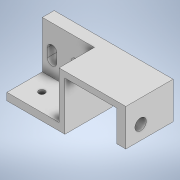
# Autodesk Inventor part: Compliant_plate
Saved by Autodesk Inventor 2022 (Build 260153000, 153)
## iProperties
Created: 2021-07-31
Part Number: Compliant_plate
Material: Generic
Document SubType Name: Modeling
Designer: exllu
Density: 1 g/cm^3
Appearance: Default
Mass: 4.01224 g
Surface Area: 39.1309 cm^2
Volume: 4.01224 cm^3
Author: exllu
Autodesk Inventor part; units mm, degrees
ref_plane "YZ Plane" through (0, 0, 0) normal (1, 0, 0) x (0, 1, 0)
ref_plane "XZ Plane" through (0, 0, 0) normal (0, 1, 0) x (-1, 0, 0)
ref_plane "XY Plane" through (0, 0, 0) normal (0, 0, 1) x (1, 0, 0)
sketch "Sketch1" plane through (0, 0, 0) normal (0, 0, 1) x (1, 0, 0)
  line L0 (0, 0) -> (49.1, 0)
  line L1 (49.1, 0) -> (49.1, 12.5)
  line L2 (49.1, 12.5) -> (0, 12.5)
  line L3 (0, 12.5) -> (0, 0)
  line L4 (0, 0) -> (49.1, 0)
  line L5 (49.1, 0) -> (49.1, 12.5)
  dimension "d0" = 49.1
  dimension "d1" = 12.5
  constraints: 12 end point, 2 horizontal, 2 parallel, 1 perpendicular, 1 vertical
  measures "d0" distance of L0.start L0.end
  measures "d1" distance of L0.end L1.end
extrude "Extrusion1" add sketch "Sketch1" along normal blind 14
sketch "Sketch2" plane through (0, 0, 0) normal (-1, 0, 0) x (0, 0, 1)
  line L0 (0, 0) -> (2, 0)
  line L1 (2, 0) -> (2, 5)
  line L2 (2, 5) -> (0, 5)
  line L3 (0, 5) -> (0, 0)
  dimension "d4" = 2
  dimension "d5" = 5
  constraints: 8 end point, 2 parallel, 1 horizontal, 1 perpendicular
  measures "d4" distance of L2.end L1.end
  measures "d5" distance of L1.end L0.end
sketch "Sketch3" plane through (0, 0, 14) normal (0, 0, 1) x (1, 0, 0)
  line L0 (0, 12.5) -> (0, 0) projected
  line L1 (49.1, 0) -> (49.1, 12.5) projected
  line L2 (0, 0) -> (49.1, 0)
  line L3 (49.1, 0) -> (47.6, 0)
  line L4 (0, 0) -> (49.1, 0) projected
  line L5 (47.6, 0) -> (47.6, 11.5)
  line L6 (49.1, 12.5) -> (0, 12.5) projected
  line L7 (47.6, 11.5) -> (19.65, 11.5)
  line L8 (19.65, 11.5) -> (19.65, 0)
  dimension "d8" = 1.5
  dimension "d9" = 11.5
  dimension "d10" = 27.95
  constraints: 10 end point, 3 perpendicular, 2 point on line, 1 horizontal
  measures "d8" distance of L1.start L3.end
  measures "d9" distance of L3.end L5.end
  measures "d10" distance of L5.end L7.end
extrude "Extrusion3" cut sketch "Sketch3" against normal blind 13 contours L8 L7 L5 L2
sketch "Sketch4" plane through (0, 0, 14) normal (-1, 0, 0) x (0, 0, 1)
  line L0 (0, 12.5) -> (0, 0) projected
  line L1 (0, 0) -> (0, 2)
  line L2 (0, 2) -> (0, 12.5)
  line L3 (0, 2) -> (-10, 2)
  line L4 (-12, 5) -> (-12, 0) projected
  line L5 (-10, 2) -> (-10, 12.5)
  line L6 (-14, 12.5) -> (0, 12.5) projected
  line L7 (-10, 12.5) -> (0, 12.5)
  point P0 (-14, 0)
  dimension "d13" = 2
  dimension "d14" = 10
  constraints: 10 end point, 2 collinear, 1 parallel, 1 perpendicular, 1 point on line
  measures "d13" distance of L0.end L1.end
  measures "d14" distance of L1.end L3.end
extrude "Extrusion4" cut sketch "Sketch4" against normal blind 17.65
sketch "Sketch5" plane through (0, 2, 14) normal (0, 1, 0) x (1, 0, 0)
  line L0 (17.65, 0) -> (0, 0) projected
  line L1 (0, 0) -> (5.825, 0)
  line L2 (5.825, 0) -> (5.825, 6)
  line L3 (5.825, 6) -> (13.825, 6)
  circle A0 centre (5.825, 6) radius 1.05
  circle A1 centre (13.825, 6) radius 1.05
  point P0 (0, 14)
  dimension "d18" = 5.825
  dimension "d19" = 6
  dimension "d20" = 8
  dimension "d21" = 2.1
  dimension "d22" = 2.1
  constraints: 6 end point, 4 coincident, 2 centre point, 1 horizontal, 1 perpendicular, 1 point on line
  measures "d18" distance of L0.end L1.end
  measures "d19" distance of L1.end L2.end
  measures "d20" distance of L2.end L3.end
  measures "d21" diameter of A0
  measures "d22" diameter of A1
hole "Hole1" at (5.825, 2, 8) at (13.825, 2, 8) direction (0, -1, 0) diameter 2.1 depth 20 tip angle 118
sketch "Sketch6" plane through (0, 0, 0) normal (0, 0, -1) x (-1, 0, 0)
  line L0 (0, 12.5) -> (0, 8.5)
  line L1 (0, 8.5) -> (-3.3, 8.5)
  line L2 (-4.9, 8.5) -> (-11.3, 8.5)
  line L3 (-12.9, 8.5) -> (-28.3, 8.5)
  line L4 (-28.3, 9.8) -> (-28.3, 10.5)
  line L5 (-28.3, 9.2) -> (-28.3, 7.5)
  line L6 (-11.3, 8.5) -> (-11.3, 10.5)
  line L7 (-11.3, 10.5) -> (-11.3, 7.5)
  line L8 (-3.3, 8.5) -> (-3.3, 9.1)
  line L9 (-3.3, 10.5) -> (-3.3, 7.5)
  arc A0 (-29.9, 7.5) -> (-26.7, 7.5) centre (-28.3, 7.5) ccw
  arc A1 (-4.9, 7.5) -> (-1.7, 7.5) centre (-3.3, 7.5) ccw
  arc A2 (-1.7, 10.5) -> (-4.9, 10.5) centre (-3.3, 10.5) ccw
  line L10 (-26.7, 10.5) -> (-26.7, 7.5)
  line L11 (-29.9, 7.5) -> (-29.9, 10.5)
  line L12 (-12.9, 10.5) -> (-12.9, 7.5)
  line L13 (-9.7, 7.5) -> (-9.7, 10.5)
  line L14 (-4.9, 10.5) -> (-4.9, 7.5)
  line L15 (-1.7, 7.5) -> (-1.7, 10.5)
  arc A3 (-12.9, 7.5) -> (-9.7, 7.5) centre (-11.3, 7.5) ccw
  arc A4 (-9.7, 10.5) -> (-12.9, 10.5) centre (-11.3, 10.5) ccw
  arc A5 (-26.7, 10.5) -> (-29.9, 10.5) centre (-28.3, 10.5) ccw
  arc A6 (-29.1307, 9.5) -> (-28.3, 9.2) centre (-28.3, 10.5) ccw
  point P0 (0, 0)
  dimension "d30" = 4
  dimension "d31" = 3.3
  dimension "d32" = 8
  dimension "d33" = 17
  dimension "d47" = 2
  dimension "d48" = 1
  dimension "d49" = 2
  dimension "d50" = 3
  dimension "d51" = 2
  dimension "d52" = 3
  dimension "d53" = 3.2
  dimension "d55" = 3.2
  dimension "d56" = 3.2
  dimension "d134" = 1.6
  constraints: 32 end point, 15 point on circle, 9 coincident, 9 tangent, 7 centre point, 6 point on line, 4 vertical, 1 perpendicular
  measures "d30" distance of L0.start L0.end
  measures "d31" distance of L0.end L1.end
  measures "d32" distance of L1.end L2.end
  measures "d33" distance of L2.end L3.end
  measures "d47" distance of point (-28.3, 8.5) L4.end
  measures "d48" distance of point (-28.3, 8.5) L5.end
  measures "d49" distance of L6.start L6.end
  measures "d50" distance of L6.end L7.end
  measures "d51" distance of L8.start L9.start
  measures "d52" distance of L9.start L9.end
  measures "d53" diameter of A0
  measures "d55" diameter of A1
  measures "d56" diameter of A2
  measures "d134" radius of A4
sketch "Sketch7" plane through (0, 0, 14) normal (0, 0, 1) x (1, 0, 0)
  line L0 (0, 12.5) -> (0, 0) projected
  line L1 (19.65, 0) -> (19.65, 11.5) projected
  line L2 (0, 0) -> (19.65, 0)
  line L3 (19.65, 0) -> (19.65, 2)
  line L4 (19.65, 2) -> (0, 2)
  line L5 (0, 2) -> (0, 0)
  line L6 (17.65, 12.5) -> (15.65, 12.5) projected
  line L7 (19.65, 2) -> (17.65, 2)
  line L8 (17.65, 2) -> (17.65, 12.5)
  line L9 (17.65, 12.5) -> (19.65, 12.5)
  line L10 (19.65, 12.5) -> (19.65, 2)
  line L11 (49.1, 0) -> (49.1, 12.5) projected
  line L12 (17.65, 12.5) -> (49.1, 12.5)
  line L13 (49.1, 12.5) -> (49.1, 11.5)
  line L14 (47.6, 11.5) -> (19.65, 11.5)
  line L15 (17.65, 11.5) -> (17.65, 12.5)
  line L16 (47.6, 11.5) -> (47.6, 0) projected
  line L17 (47.6, 11.5) -> (47.6, 0)
  line L18 (47.6, 0) -> (49.1, 0)
  line L19 (49.1, 0) -> (49.1, 11.5)
  dimension "d41" = 2
  constraints: 30 end point, 7 parallel, 3 horizontal, 3 perpendicular, 3 point on line
  measures "d41" distance of L3.end L2.end
extrude "Extrusion5" add sketch "Sketch7" along normal blind 2
sketch "Sketch9" plane through (0, 0, 0) normal (-1, 0, 0) x (0, 0, 1)
  line L0 (0, 0) -> (16, 0) projected
  line L1 (1, 0) -> (1, 11.5) projected
  line L2 (0, 0) -> (1, 0)
  line L3 (1, 0) -> (1, 4)
  line L4 (1, 4) -> (0, 4)
  line L5 (0, 4) -> (0, 0)
  dimension "d44" = 4
  constraints: 8 end point, 2 parallel, 1 horizontal, 1 perpendicular, 1 point on line
  measures "d44" distance of L3.end L2.end
extrude "Extrusion6" cut sketch "Sketch9" against normal blind 100
sketch "Sketch11" plane through (0, 2, 4) normal (-1, 0, 0) x (0, 0, 1)
  line L0 (0, 0) -> (0, 10.5) projected
  line L1 (0, 0) -> (0, 2)
  line L2 (-4, 10.5) -> (-4, 2) projected
  line L3 (0, 2) -> (-4, 2)
  line L4 (-4, 2) -> (-6, 2)
  line L5 (-6, 2) -> (-6, 10.5)
  line L6 (-4, 10.5) -> (0, 10.5) projected
  line L7 (-6, 10.5) -> (-4, 10.5)
  line L8 (-4, 10.5) -> (-4, 2)
  point P0 (-4, -2)
  dimension "d61" = 2
  dimension "d62" = 4
  dimension "d63" = 2
  constraints: 12 end point, 2 perpendicular, 2 point on line
  measures "d61" distance of L0.start L1.end
  measures "d62" distance of L1.end L2.end
  measures "d63" distance of L2.end L4.end
extrude "Extrusion8" add sketch "Sketch11" against normal blind 49.1 contours L4 L5 L7 L2
extrude "Extrusion7" cut sketch "Sketch6" along normal blind 100 and the other way blind 50
sketch "Sketch12" plane through (0, 2, 4) normal (-1, 0, 0) x (0, 0, 1)
  line L0 (0, 0) -> (0, 10.5) projected
  line L1 (0, 0) -> (-3, 0)
  line L2 (-3, -2) -> (-3, 2) projected
  line L3 (-3, -2) -> (12, -2) projected
  line L4 (-3, -2) -> (-6, -2)
  line L5 (-3, 2) -> (-6, 2) projected
  line L6 (-6, -2) -> (-6, 2)
  line L7 (-6, 2) -> (-3, 2)
  line L8 (-3, 2) -> (-3, -2)
  point P0 (-4, -2)
  dimension "d68" = 3
  dimension "d69" = 4
  dimension "d70" = 90
  constraints: 10 end point, 1 horizontal, 1 midpoint, 1 perpendicular
  measures "d68" distance of L2.start L4.end
  measures "d69" distance of L4.end L5.end
  measures "d70" angle of L4 L6
extrude "Extrusion9" add sketch "Sketch12" against normal blind 49.1
sketch "Sketch13" plane through (47.6, 0, 1) normal (-1, 0, 0) x (0, 0, 1)
  line L0 (15, 0) -> (0, 0) projected
  line L1 (0, 11.5) -> (0, 0) projected
  line L2 (0, 0) -> (0, 11.5)
  line L3 (15, 11.5) -> (0, 11.5) projected
  line L4 (0, 11.5) -> (15, 11.5)
  line L5 (15, 11.5) -> (15, 0)
  line L6 (15, 0) -> (0, 0)
  point P0 (-1, 0)
  constraints: 8 end point, 2 collinear, 2 perpendicular
extrude "Extrusion10" add sketch "Sketch13" along normal blind 1
sketch "Sketch14" plane through (49.1, 0, 16) normal (1, 0, 0) x (0, 0, -1)
  line L0 (15, 0) -> (0, 0) projected
  line L1 (18, 12.5) -> (0, 12.5) projected
  line L2 (0, 0) -> (18, 0)
  line L3 (18, 0) -> (18, 12.5)
  line L4 (18, 12.5) -> (0, 12.5)
  line L5 (0, 12.5) -> (0, 0)
  point P0 (16, 0)
  constraints: 8 end point, 2 parallel, 1 horizontal, 1 perpendicular
extrude "Extrusion11" cut sketch "Sketch14" against normal blind 12.3
sketch "Sketch15" plane through (36.8, 0, 16) normal (1, 0, 0) x (0, 0, -1)
  line L0 (18, 12.5) -> (18, 0) projected
  line L1 (15, 0) -> (0, 0) projected
  line L2 (18, 12.5) -> (0, 12.5)
  line L3 (0, 12.5) -> (0, 0)
  line L4 (0, 0) -> (18, 0)
  line L5 (18, 0) -> (18, 12.5)
  point P0 (16, 0)
  point P1 (18, 0)
  constraints: 8 end point, 2 parallel, 1 horizontal, 1 perpendicular
extrude "Extrusion12" add sketch "Sketch15" along normal blind 2.5
sketch "Sketch17" plane through (0, 0, -2) normal (0, -1, 0) x (1, 0, 0)
  line L0 (39.3, 0) -> (39.3, 18) projected
  line L1 (39.3, 0) -> (39.3, 16)
  line L2 (39.3, 16) -> (36.8, 16)
  line L3 (36.8, 3) -> (36.8, 18) projected
  line L4 (36.8, 16) -> (36.8, 3)
  line L5 (19.65, 3) -> (36.8, 3) projected
  line L6 (36.8, 3) -> (19.65, 3)
  line L7 (19.65, 3) -> (19.65, 0)
  line L8 (0, 0) -> (39.3, 0) projected
  line L9 (19.65, 0) -> (39.3, 0)
  point P0 (0, 2)
  constraints: 12 end point, 3 collinear, 3 perpendicular
extrude "Extrusion14" cut sketch "Sketch17" against normal blind 5
sketch "Sketch18" plane through (36.8, 0, 16) normal (0, -1, 0) x (1, 0, 0)
  line L0 (2.5, 0) -> (-19.15, 0) projected
  line L1 (2.5, 0) -> (0, 0)
  line L2 (0, 0) -> (0, -2)
  line L3 (0, -2) -> (2.5, -2)
  line L4 (2.5, -2) -> (2.5, 0)
  point P0 (-36.8, -16)
  dimension "d84" = 2.5
  dimension "d85" = 2
  constraints: 8 end point, 2 parallel, 1 horizontal, 1 perpendicular
  measures "d84" distance of L3.end L2.end
  measures "d85" distance of L2.end L1.end
extrude "Extrusion15" cut sketch "Sketch18" against normal blind 5
sketch "Sketch19" plane through (19.65, 11.5, 1) normal (0, -1, 0) x (1, 0, 0)
  line L0 (0, 15) -> (0, 0) projected
  line L1 (0, 0) -> (0, 15)
  line L2 (0, 15) -> (17.15, 15)
  line L3 (19.65, 15) -> (-2, 15) projected
  line L4 (17.15, 15) -> (17.15, 0)
  line L5 (17.15, 0) -> (0, 0)
  point P0 (-19.65, -1)
  point P1 (0, 0)
  dimension "d88" = 17.15
  dimension "d89" = 15
  constraints: 8 end point, 2 perpendicular, 2 point on line, 1 collinear
  measures "d88" distance of L0.start L2.end
  measures "d89" distance of L2.end L4.end
extrude "Extrusion16" cut sketch "Sketch19" against normal blind 5
sketch "Sketch20" plane through (0, 12.5, 4) normal (0, 1, 0) x (1, 0, 0)
  line L0 (0, 6) -> (0, -12) projected
  line L1 (0, 6) -> (0, 0)
  line L2 (0, 6) -> (39.3, 6) projected
  line L3 (0, 6) -> (39.3, 6)
  line L4 (39.3, -12) -> (39.3, 6) projected
  line L5 (39.3, 6) -> (39.3, -12)
  line L6 (39.3, -12) -> (36.8, -12) projected
  line L7 (39.3, -12) -> (36.8, -12)
  line L8 (36.8, -12) -> (36.8, 3)
  line L9 (36.8, 3) -> (19.65, 3)
  line L10 (19.65, -12) -> (19.65, 3) projected
  line L11 (19.65, 3) -> (19.65, -12)
  line L12 (17.65, -12) -> (17.65, 0) projected
  line L13 (19.65, -12) -> (17.65, -12)
  line L14 (17.65, -12) -> (17.65, 0)
  line L15 (17.65, 0) -> (17.65, 6)
  point P0 (0, 4)
  dimension "d92" = 6
  constraints: 20 end point, 4 collinear, 3 perpendicular, 3 point on line, 1 horizontal
  measures "d92" distance of L0.start L1.end
extrude "Extrusion17" add sketch "Sketch20" along normal blind 4
sketch "Sketch21" plane through (0, 12.5, 4) normal (0, 1, 0) x (1, 0, 0)
  line L0 (0, -12) -> (0, 0) projected
  line L1 (0, 0) -> (17.65, 0)
  line L2 (17.65, 0) -> (17.65, 6)
  line L3 (17.65, 6) -> (0, 6)
  line L4 (0, 6) -> (0, 0)
  point P0 (0, 4)
  constraints: 8 end point, 2 parallel, 1 horizontal, 1 perpendicular
extrude "Extrusion18" add sketch "Sketch21" along normal blind 4
sketch "Sketch22" plane through (0, 16.5, 4) normal (0, 1, 0) x (1, 0, 0)
  line L0 (0, 6) -> (0, 0) projected
  line L1 (0, 0) -> (36.92, 0)
  line L2 (19.65, 3) -> (36.8, 3) projected
  line L3 (36.8, 3) -> (36.8, 0)
  line L4 (36.8, 3) -> (36.8, -12) projected
  line L5 (36.8, 0) -> (36.3, 0)
  line L6 (36.3, 0) -> (36.3, 3)
  point P0 (0, 4)
  dimension "d97" = 3
  dimension "d98" = 0.5
  constraints: 8 end point, 2 point on line, 1 horizontal, 1 perpendicular
  measures "d97" distance of L2.end L3.end
  measures "d98" distance of L3.end L5.end
extrude "Extrusion19" add sketch "Sketch22" against normal blind 11.5
sketch "Sketch23" plane through (36.8, 0, 16) normal (-1, 0, 0) x (0, 0, 1)
  line L0 (0, 0) -> (0, 5)
  line L1 (-12, 5) -> (0, 5) projected
  line L2 (0, 5) -> (-12, 5)
  line L3 (-12, 16.5) -> (-12, 5) projected
  line L4 (-12, 5) -> (-12, 16.5)
  line L5 (-12, 16.5) -> (0, 16.5)
  line L6 (0, 16.5) -> (0, 5)
  line L7 (0, 5) -> (0, 16.5) projected
  line L8 (0, 10.75) -> (-7, 10.75)
  circle A0 centre (-7, 10.75) radius 1.9304
  point P0 (-16, 0)
  dimension "d101" = 5
  dimension "d102" = 12
  dimension "d103" = 7
  dimension "d104" = 3.8608
  constraints: 12 end point, 3 perpendicular, 1 centre point, 1 coincident, 1 collinear, 1 horizontal, 1 midpoint, 1 vertical
  measures "d101" distance of L0.start L0.end
  measures "d102" distance of L0.end L1.start
  measures "d103" distance of L8.start L8.end
  measures "d104" diameter of A0
sketch "Sketch24" plane through (0, 16.5, 4) normal (0, 1, 0) x (1, 0, 0)
  line L0 (39.3, -12) -> (39.3, 6) projected
  line L1 (39.3, -12) -> (36.3, -12)
  line L2 (36.8, -12) -> (39.3, -12) projected
  line L3 (36.3, -12) -> (36.3, 0)
  line L4 (36.3, 0) -> (36.8, 0) projected
  line L5 (36.8, 0) -> (36.8, -12) projected
  line L6 (36.8, 0) -> (36.8, -12)
  point P0 (0, 4)
  dimension "d107" = 3
  constraints: 6 end point, 2 collinear, 1 perpendicular, 1 point on line
  measures "d107" distance of L0.start L1.end
extrude "Extrusion21" add sketch "Sketch24" against normal blind 11.5
extrude "Extrusion22" cut sketch "Sketch23" along normal mid plane 11.5 contours A0
sketch "Sketch25" plane through (0, 16.5, 4) normal (0, 1, 0) x (1, 0, 0)
  line L0 (17.65, -12) -> (0, -12) projected
  line L1 (39.3, 6) -> (0, 6) projected
  line L2 (0, -12) -> (39.3, -12)
  line L3 (39.3, -12) -> (39.3, 6)
  line L4 (39.3, 6) -> (0, 6)
  line L5 (0, 6) -> (0, -12)
  line L6 (0, 0) -> (17.65, 0) projected
  line L7 (17.65, 0) -> (0, 0)
  line L8 (0, 0) -> (0, -12)
  line L9 (0, -12) -> (17.65, -12)
  line L10 (17.65, -12) -> (17.65, 0)
  point P0 (0, 4)
  constraints: 16 end point, 4 parallel, 2 horizontal, 2 perpendicular
extrude "Extrusion23" add sketch "Sketch25" along normal blind 2 contours L10 L6 L5 L1 L3 L2
sketch "Sketch26" plane through (0, 0, 16) normal (0, 0, 1) x (1, 0, 0)
  line L0 (0, 18.5) -> (0, 0) projected
  line L1 (19.65, 0) -> (19.65, 16.5) projected
  line L2 (0, 0) -> (19.65, 0)
  line L3 (19.65, 5) -> (19.65, 16.5) projected
  line L4 (19.65, 0) -> (19.65, 16.5)
  line L5 (19.65, 16.5) -> (36.3, 16.5) projected
  line L6 (19.65, 16.5) -> (36.3, 16.5)
  line L7 (36.3, 16.5) -> (36.3, 5) projected
  line L8 (36.3, 16.5) -> (36.3, 5)
  line L9 (39.3, 5) -> (19.65, 5) projected
  line L10 (36.3, 5) -> (39.3, 5)
  line L11 (39.3, 18.5) -> (0, 18.5) projected
  line L12 (39.3, 5) -> (39.3, 18.5)
  line L13 (39.3, 18.5) -> (17.65, 18.5)
  line L14 (0, 2) -> (17.65, 2) projected
  line L15 (0, 0) -> (0, 2)
  line L16 (0, 2) -> (17.65, 2)
  line L17 (0, 2) -> (17.65, 2)
  line L18 (17.65, 2) -> (17.65, 18.5)
  line L19 (17.65, 18.5) -> (0, 18.5)
  line L20 (0, 18.5) -> (0, 2)
  dimension "d114" = 3
  dimension "d115" = 21.65
  constraints: 26 end point, 4 perpendicular, 3 collinear, 2 horizontal, 2 parallel, 1 point on line, 1 vertical
  measures "d114" distance of L7.end L9.start
  measures "d115" distance of L11.start L13.end
extrude "Extrusion24" cut sketch "Sketch26" against normal blind 2 contours L14 L18 L11 L12 L9 L7 L5 L1 L2 L0
sketch "Sketch27" plane through (39.3, 0, 16) normal (1, 0, 0) x (0, 0, -1)
  line L0 (18, 18.5) -> (18, 0) projected
  line L1 (18, 0) -> (18, 5)
  line L2 (2, 5) -> (15, 5) projected
  line L3 (18, 5) -> (2, 5)
  line L4 (2, 18.5) -> (18, 18.5) projected
  line L5 (2, 5) -> (2, 18.5)
  line L6 (2, 18.5) -> (18, 18.5)
  line L7 (18, 18.5) -> (18, 5)
  circle A0 centre (7, 10.75) radius 1.9304 projected
  circle A1 centre (7, 10.75) radius 1.5
  point P0 (16, 0)
  dimension "d118" = 5
  dimension "d119" = 16
  constraints: 10 end point, 2 perpendicular, 1 centre point, 1 coincident, 1 collinear, 1 point on line
  measures "d118" distance of L0.end L1.end
  measures "d119" distance of L1.end L2.start
extrude "Extrusion25" add sketch "Sketch27" along normal blind 1 contours L0 L3 L2 L5 L4
sketch "Sketch28" plane through (36.3, 5, 1) normal (-1, 0, 0) x (0, 0, 1)
  line L0 (0, 0) -> (0, 11.5) projected
  line L1 (0, 0) -> (0, 11.5)
  line L2 (0, 11.5) -> (13, 11.5) projected
  line L3 (0, 11.5) -> (13, 11.5)
  line L4 (13, 11.5) -> (13, 0)
  line L5 (13, 0) -> (0, 0) projected
  line L6 (13, 0) -> (0, 0)
  circle A0 centre (8, 5.75) radius 1.9304 projected
  circle A1 centre (8, 5.75) radius 1.5
  point P0 (-1, -5)
  dimension "d122" = 11.5
  constraints: 8 end point, 3 collinear, 1 centre point, 1 coincident, 1 perpendicular
  measures "d122" distance of L0.start L0.end
extrude "Extrusion26" cut sketch "Sketch28" against normal blind 1 contours L0 L2 L4 L5
sketch "Sketch29" plane through (0, 5, -2) normal (0, -1, 0) x (1, 0, 0)
  line L0 (19.65, 0) -> (19.65, 3) projected
  line L1 (19.65, 0) -> (19.65, 3)
  line L2 (19.65, 3) -> (19.65, 2)
  line L3 (19.65, 2) -> (37.4623, 2)
  line L4 (19.65, 3) -> (37.3, 3) projected
  line L5 (37.3, 3) -> (37.3, 1.7723)
  line L6 (37.3, 3) -> (19.65, 3)
  point P0 (0, 2)
  point P1 (37.3, 2)
  dimension "d125" = 1
  constraints: 10 end point, 2 collinear, 1 perpendicular, 1 point on line, 1 vertical
  measures "d125" distance of L0.end L2.end
extrude "Extrusion27" cut sketch "Sketch29" against normal blind 11.5
sketch "Sketch30" plane through (0, 2, 4) normal (0, 1, 0) x (1, 0, 0)
  line L0 (0, 0) -> (17.65, 0) projected
  line L1 (17.65, -10) -> (17.65, 0) projected
  line L2 (0, 0) -> (17.65, 0)
  line L3 (17.65, 0) -> (17.65, -10)
  line L4 (17.65, -10) -> (0, -10)
  line L5 (0, -10) -> (0, 0)
  circle A0 centre (5.825, -4) radius 1.05 projected
  circle A1 centre (5.825, -4) radius 1.05
  circle A2 centre (13.825, -4) radius 1.05 projected
  circle A3 centre (13.825, -4) radius 1.05
  point P0 (0, 4)
  constraints: 8 end point, 2 centre point, 2 coincident, 2 parallel, 1 horizontal, 1 perpendicular
extrude "Extrusion29" add sketch "Sketch30" along normal blind 0.3
sketch "Sketch31" plane through (0, 18.5, 4) normal (0, 0, 1) x (1, 0, 0)
  line L0 (0, 0) -> (0, -18.5) projected
  line L1 (17.65, 0) -> (17.65, -16.2) projected
  line L2 (0, 0) -> (17.65, 0)
  line L3 (17.65, 0) -> (17.65, -16.2)
  line L4 (17.65, -16.2) -> (0, -16.2)
  line L5 (0, -16.2) -> (0, 0)
  constraints: 8 end point, 2 parallel, 1 horizontal, 1 perpendicular
extrude "Extrusion30" cut sketch "Sketch31" against normal blind 2
sketch "Sketch32" plane through (0, 2.3, 4) normal (0, 1, 0) x (1, 0, 0)
  line L0 (0, 2) -> (17.65, 2) projected
  line L1 (0, -10) -> (17.65, -10) projected
  line L2 (0, 2) -> (17.65, 2)
  line L3 (17.65, 2) -> (17.65, -10)
  line L4 (17.65, -10) -> (0, -10)
  line L5 (0, -10) -> (0, 2)
  circle A0 centre (5.825, -4) radius 1.05 projected
  circle A1 centre (5.825, -4) radius 1.05
  circle A2 centre (13.825, -4) radius 1.05 projected
  circle A3 centre (13.825, -4) radius 1.05
  point P0 (0, 4)
  point P1 (17.65, 2)
  constraints: 8 end point, 2 centre point, 2 coincident, 2 parallel, 1 horizontal, 1 perpendicular
extrude "Extrusion31" add sketch "Sketch32" along normal blind 0.2
sketch "Sketch33" plane through (40.3, 0, 16) normal (1, 0, 0) x (0, 0, -1)
  line L0 (2, 5) -> (18, 5) projected
  line L1 (2, 18.5) -> (2, 5) projected
  line L2 (18, 5) -> (2, 5)
  line L3 (2, 5) -> (2, 6)
  line L4 (2, 6) -> (18, 6)
  line L5 (18, 6) -> (18, 5)
  point P0 (16, 0)
  dimension "d137" = 1
  constraints: 8 end point, 2 parallel, 1 horizontal, 1 perpendicular, 1 point on line
  measures "d137" distance of L2.end L3.end
extrude "Extrusion32" cut sketch "Sketch33" against normal blind 3
chamfer "Chamfer1" distance 1 angle 45 1 edges at (37.3, 5, -1)
body "Solid1"
